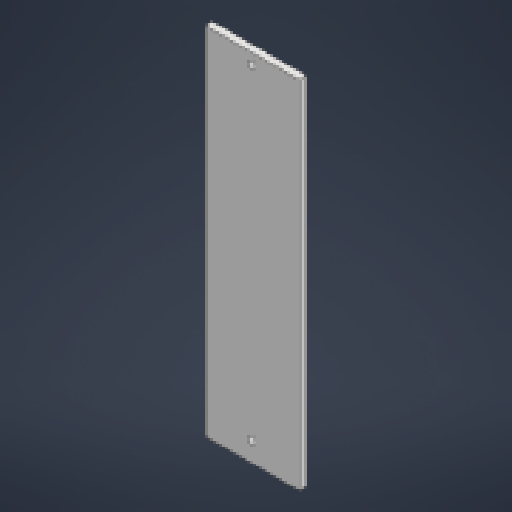
# Autodesk Inventor part: ff-hta
Saved by Autodesk Inventor 2026.1 (Build 301233020, 233B)
## iProperties
Created: 2026-03-20
Part Number: ff-hta
Material: 一般
Document SubType Name: Modeling
Designer: kamada
Density: 1 g/cm^3
Appearance: 既定
Author: kamada
Autodesk Inventor part; units mm, degrees
ref_plane "YZ Plane" through (0, 0, 0) normal (1, 0, 0) x (0, 1, 0)
ref_plane "XZ Plane" through (0, 0, 0) normal (0, 1, 0) x (-1, 0, 0)
ref_plane "XY Plane" through (0, 0, 0) normal (0, 0, 1) x (1, 0, 0)
sketch "スケッチ1" plane through (0, 0, 0) normal (0, 0, 1) x (1, 0, 0)
  circle A0 centre (-0.0006, 1.5287) radius 1 projected
  line L0 (-13.25, 3.9997) -> (13.25, 3.9997) projected
  line L1 (-13.25, -3.9997) -> (-13.25, 3.9997) projected
  line L2 (13.25, -3.9997) -> (-13.25, -3.9997) projected
  line L3 (13.25, 3.9997) -> (13.25, -3.9997) projected
  circle A1 centre (0, 91.051) radius 1 projected
  line L4 (13.25, 88.9997) -> (-13.25, 88.9997) projected
  line L5 (13.25, 93.9997) -> (13.25, 88.9997) projected
  line L6 (-13.25, 93.9997) -> (13.25, 93.9997) projected
  line L7 (-13.25, 88.9997) -> (-13.25, 93.9997) projected
  line L8 (12.95, -3.9997) -> (-12.95, -3.9997)
  line L9 (-12.95, -3.9997) -> (-12.95, 93.9997)
  line L10 (-12.95, 93.9997) -> (12.95, 93.9997)
  line L11 (12.95, 93.9997) -> (12.95, -3.9997)
  point P0 (0, 0)
  point P1 (0, -3.9997)
  point P2 (0, -3.9997)
  dimension "d0" = 0.3
  constraints: 8 end point, 2 midpoint, 2 parallel, 2 point on line, 1 coincident, 1 horizontal, 1 perpendicular
  measures "d0" distance between parallel lines of L1 L9
extrude "押し出し1" add sketch "スケッチ1" along normal blind 2 contours L9 L4 L11 L0 | L0 L11 L2 L9 | L9 L6 L11 L4
